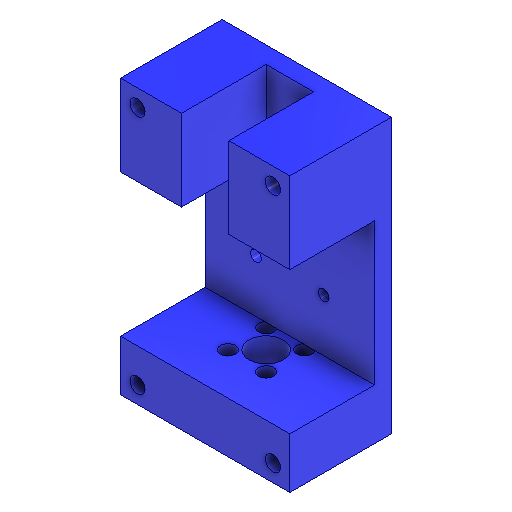
# Autodesk Inventor part: y_slider_bracket
Saved by Autodesk Inventor 2026.1 (Build 301233000, 233)
## iProperties
Created: 2025-01-02
Part Number: y_slider_bracket
Material: PC/ABS Plastic
Document SubType Name: Modeling
Designer: drago
Density: 1.24303 g/cm^3
Appearance: Blue - Wall Paint - Glossy
Author: drago
Autodesk Inventor part; units mm, degrees
ref_plane "YZ Plane" through (0, 0, 0) normal (1, 0, 0) x (0, 1, 0)
ref_plane "Work Plane1" through (-22.1363, -57.0374, 30) normal (0, 0, 1) x (1, 0, 0)
sketch "Sketch1" plane through (-22.1363, -57.0374, 30) normal (0, 0, 1) x (1, 0, 0)
  line L0 (0, 0) -> (50, 0)
  line L1 (50, 0) -> (50, 81)
  line L2 (50, 81) -> (0, 81)
  line L3 (0, 81) -> (0, 0)
  line L4 (25, 81) -> (25, 0) construction
  line L5 (0, 40.5) -> (50, 40.5) construction
  circle A0 centre (5, 76) radius 2.25
  circle A1 centre (45, 5) radius 2.25
  circle A2 centre (45, 76) radius 2.25
  circle A3 centre (5, 5) radius 2.25
  line L6 (18, 81) -> (18, 0)
  line L7 (32, 81) -> (32, 0)
  line L8 (0, 15) -> (50, 15)
  line L9 (0, 57) -> (50, 57)
  circle A4 centre (35, 30.5) radius 1.6
  circle A5 centre (15, 50.5) radius 1.6
  circle A6 centre (15, 30.5) radius 1.6
  circle A7 centre (35, 50.5) radius 1.6
  point P0 (18, 57)
  point P1 (32, 57)
  dimension "d0" = 50
  dimension "d1" = 81
  dimension "d2" = 5
  dimension "d3" = 5
  dimension "d5" = 4.5
  dimension "d27" = 14
  dimension "d28" = 24
  dimension "d29" = 15
  dimension "d30" = 20
  dimension "d31" = 20
  dimension "d32" = 3.2
  constraints: 20 end point, 9 coincident, 8 centre point, 8 point on line, 7 symmetric about line, 6 equal radius, 5 perpendicular, 4 midpoint, 2 parallel, 1 horizontal, 4 other
  measures "d0" distance of L2.end L1.end
  measures "d1" distance of L1.end L0.end
  measures "d2" distance from line of L2 point (5, 76)
  measures "d3" distance from line of L3 point (5, 76)
  measures "d5" diameter of A0
  measures "d27" distance between parallel lines of L7 L6
  measures "d28" distance between parallel lines of L2 L9
  measures "d29" distance between parallel lines of L0 L8
  measures "d30" distance of point (35, 30.5) point (35, 50.5)
  measures "d31" distance of point (35, 30.5) point (15, 30.5)
  measures "d32" diameter of A5
ref_plane "Work Plane4" through (-22.1363, -57.0374, 0) normal (0, -1, 0) x (1, 0, 0)
sketch "Sketch2" plane through (-22.1363, -57.0374, 0) normal (0, -1, 0) x (1, 0, 0)
  line L0 (0, 0) -> (50, 0)
  line L1 (50, 0) -> (50, 30)
  line L2 (50, 30) -> (0, 30)
  line L3 (0, 30) -> (0, 0)
  line L4 (25, 0) -> (25, 30) construction
  line L5 (0, 12) -> (50, 12) construction
  circle A0 centre (25, 12) radius 5.1
  circle A1 centre (30.6569, 17.6569) radius 2.25
  line L6 (25, 12) -> (30.6569, 17.6569) construction
  circle A2 centre (19.3431, 6.3431) radius 2.25
  circle A3 centre (30.6569, 6.3431) radius 2.25
  circle A4 centre (19.3431, 17.6569) radius 2.25
  dimension "d17" = 50
  dimension "d18" = 30
  dimension "d21" = 12
  dimension "d22" = 10.2
  dimension "d24" = 4.5
  dimension "d25" = 8
  dimension "d26" = 45
  constraints: 14 end point, 7 coincident, 5 centre point, 3 equal radius, 3 midpoint, 3 parallel, 3 point on line, 1 horizontal, 1 perpendicular, 5 other
  measures "d17" distance of L2.end L1.end
  measures "d18" distance of L1.end L0.end
  measures "d21" distance between parallel lines of L0 L5
  measures "d22" diameter of A0
  measures "d24" diameter of A1
  measures "d25" distance of L6.start L6.end
  measures "d26" angle of L5 L6
extrude "Extrusion1" add sketch "Sketch1" against normal blind 30 contours L3 L8 L6 L0 | L6 L8 L7 L0 | L3 L9 L6 L8 | L7 L8 L1 L0 | L6 L9 L7 L8 | L3 L2 L6 L9 | L7 L9 L1 L8 | L6 L2 L7 L9 | L7 L2 L1 L9 | A0 | A1 | A2 | A3 | A4 | A5 | A6 | A7
hole "Hole2" at (-7.1363, -6.5374, 30) at (12.8637, -6.5374, 30) at (12.8637, -26.5374, 30) at (-7.1363, -26.5374, 30) direction (0, 0, -1) diameter 3.2 end through all
hole "Hole3" at (-17.1363, 18.9626, 30) at (22.8637, 18.9626, 30) at (22.8637, -52.0374, 30) at (-17.1363, -52.0374, 30) direction (0, 0, -1) diameter 4.5 end through all
hole "Hole4" at (-2.7932, -57.0374, 17.6569) at (8.5205, -57.0374, 17.6569) at (8.5205, -57.0374, 6.3431) at (-2.7932, -57.0374, 6.3431) direction (0, 1, 0) diameter 4.5 depth 15
hole "Hole5" at (2.8637, -57.0374, 12) direction (0, 1, 0) diameter 10.2 end through all
extrude "Extrusion2" cut sketch "Sketch1" against normal blind 25 contours L3 L9 L6 L8 | L6 L9 L7 L8 | L7 L9 L1 L8 | L6 L2 L7 L9
body "Solid3"
